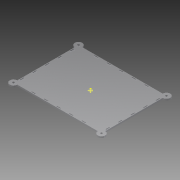
# Autodesk Inventor part: BasePlate2
Saved by Autodesk Inventor 2015 (Build 190159000, 159)
## iProperties
Created: 2014-08-06
Part Number: BasePlate2
Material: Acrylic, Clear
Document SubType Name: Modeling
Designer: Patrick Camilleri
Density: 1.19 g/cm^3
Appearance: Transparent - Clear
Mass: 654.149 g
Surface Area: 1962.87 cm^2
Volume: 549.705 cm^3
Author: Patrick Camilleri
Autodesk Inventor part; units mm, degrees
ref_plane "YZ Plane" through (0, 0, 0) normal (1, 0, 0) x (0, 1, 0)
ref_plane "XZ Plane" through (0, 0, 0) normal (0, 1, 0) x (-1, 0, 0)
ref_plane "XY Plane" through (0, 0, 0) normal (0, 0, 1) x (1, 0, 0)
sketch "Sketch1" plane through (0, 0, 0) normal (0, 0, 1) x (1, 0, 0)
  line L0 (-175, 129.3) -> (175, 129.3)
  line L1 (175, 129.3) -> (175, -129.3)
  line L2 (175, -129.3) -> (-175, -129.3)
  line L3 (-175, -129.3) -> (-175, 129.3)
  line L4 (-175, 129.3) -> (175, -129.3) construction
  line L5 (175, 129.3) -> (-175, -129.3) construction
  circle A0 centre (-175, -129.3) radius 15
  circle A1 centre (-175, 129.3) radius 15
  circle A2 centre (175, 129.3) radius 15
  circle A3 centre (175, -129.3) radius 15
  point P0 (0, 0)
  dimension "d0" = 350
  dimension "d1" = 258.6
  dimension "d2" = 30
  dimension "d3" = 30
  dimension "d4" = 30
  dimension "d5" = 30
  constraints: 12 end point, 4 centre point, 4 coincident, 2 midpoint, 2 parallel, 1 horizontal, 1 perpendicular
  measures "d0" distance of L1.end L2.end
  measures "d1" distance of L0.end L1.end
  measures "d2" diameter of A0
  measures "d3" diameter of A1
  measures "d4" diameter of A2
  measures "d5" diameter of A3
extrude "Extrusion1" add sketch "Sketch1" along normal blind 6
hole "Hole1" at (-175, 129.3, 6) direction (0, 0, -1) diameter 8 end through all
mirror "Mirror1" about plane through (0, 0, 0) normal (1, 0, 0) of "Hole1"
mirror "Mirror2" about plane through (0, 0, 0) normal (0, 1, 0) of "Hole1", "Mirror1"
sketch "Sketch2" plane through (0, 0, 6) normal (0, 0, 1) x (1, 0, 0)
  line L0 (160, 129.3) -> (-160, 129.3) projected
  line L1 (-175, 114.3) -> (-175, -114.3) projected
  line L2 (-160, -129.3) -> (160, -129.3) projected
  line L3 (175, -114.3) -> (175, 114.3) projected
  line L4 (-170.5, 124.8) -> (170.5, 124.8) construction
  line L5 (170.5, 124.8) -> (170.5, -124.8) construction
  line L6 (170.5, -124.8) -> (-170.5, -124.8) construction
  line L7 (-170.5, -124.8) -> (-170.5, 124.8) construction
  line L8 (-170.5, 124.8) -> (170.5, -124.8) construction
  line L9 (170.5, 124.8) -> (-170.5, -124.8) construction
  line L10 (-7.5, 126.3) -> (7.5, 126.3)
  line L11 (7.5, 126.3) -> (7.5, 123.3)
  line L12 (7.5, 123.3) -> (-7.5, 123.3)
  line L13 (-7.5, 123.3) -> (-7.5, 126.3)
  line L14 (-7.5, 126.3) -> (7.5, 123.3) construction
  line L15 (7.5, 126.3) -> (-7.5, 123.3) construction
  line L16 (-57.5, 126.3) -> (-42.5, 126.3)
  line L17 (-42.5, 126.3) -> (-42.5, 123.3)
  line L18 (-42.5, 123.3) -> (-57.5, 123.3)
  line L19 (-57.5, 123.3) -> (-57.5, 126.3)
  line L20 (-107.5, 126.3) -> (-92.5, 126.3)
  line L21 (-92.5, 126.3) -> (-92.5, 123.3)
  line L22 (-92.5, 123.3) -> (-107.5, 123.3)
  line L23 (-107.5, 123.3) -> (-107.5, 126.3)
  line L24 (42.5, 126.3) -> (57.5, 126.3)
  line L25 (57.5, 126.3) -> (57.5, 123.3)
  line L26 (57.5, 123.3) -> (42.5, 123.3)
  line L27 (42.5, 123.3) -> (42.5, 126.3)
  line L28 (92.5, 126.3) -> (107.5, 126.3)
  line L29 (107.5, 126.3) -> (107.5, 123.3)
  line L30 (107.5, 123.3) -> (92.5, 123.3)
  line L31 (92.5, 123.3) -> (92.5, 126.3)
  line L32 (7.5, -126.3) -> (-7.5, -126.3)
  line L33 (-7.5, -126.3) -> (-7.5, -123.3)
  line L34 (-7.5, -123.3) -> (7.5, -123.3)
  line L35 (7.5, -123.3) -> (7.5, -126.3)
  line L36 (7.5, -126.3) -> (-7.5, -123.3) construction
  line L37 (-7.5, -126.3) -> (7.5, -123.3) construction
  line L38 (57.5, -126.3) -> (42.5, -126.3)
  line L39 (42.5, -126.3) -> (42.5, -123.3)
  line L40 (42.5, -123.3) -> (57.5, -123.3)
  line L41 (57.5, -123.3) -> (57.5, -126.3)
  line L42 (107.5, -126.3) -> (92.5, -126.3)
  line L43 (92.5, -126.3) -> (92.5, -123.3)
  line L44 (92.5, -123.3) -> (107.5, -123.3)
  line L45 (107.5, -123.3) -> (107.5, -126.3)
  line L46 (120.5, -124.8) -> (-220.5, -124.8) construction
  line L47 (-42.5, -126.3) -> (-57.5, -126.3)
  line L48 (-57.5, -126.3) -> (-57.5, -123.3)
  line L49 (-57.5, -123.3) -> (-42.5, -123.3)
  line L50 (-42.5, -123.3) -> (-42.5, -126.3)
  line L51 (70.5, -124.8) -> (-270.5, -124.8) construction
  line L52 (-92.5, -126.3) -> (-107.5, -126.3)
  line L53 (-107.5, -126.3) -> (-107.5, -123.3)
  line L54 (-107.5, -123.3) -> (-92.5, -123.3)
  line L55 (-92.5, -123.3) -> (-92.5, -126.3)
  line L56 (-172, 7.5) -> (-169, 7.5)
  line L57 (-169, 7.5) -> (-169, -7.5)
  line L58 (-169, -7.5) -> (-172, -7.5)
  line L59 (-172, -7.5) -> (-172, 7.5)
  line L60 (-172, 7.5) -> (-169, -7.5) construction
  line L61 (-169, 7.5) -> (-172, -7.5) construction
  line L62 (-172, -42.5) -> (-169, -42.5)
  line L63 (-169, -42.5) -> (-169, -57.5)
  line L64 (-169, -57.5) -> (-172, -57.5)
  line L65 (-172, -57.5) -> (-172, -42.5)
  line L66 (-172, -92.5) -> (-169, -92.5)
  line L67 (-169, -92.5) -> (-169, -107.5)
  line L68 (-169, -107.5) -> (-172, -107.5)
  line L69 (-172, -107.5) -> (-172, -92.5)
  line L70 (-172, 57.5) -> (-169, 57.5)
  line L71 (-169, 57.5) -> (-169, 42.5)
  line L72 (-169, 42.5) -> (-172, 42.5)
  line L73 (-172, 42.5) -> (-172, 57.5)
  line L74 (-172, 107.5) -> (-169, 107.5)
  line L75 (-169, 107.5) -> (-169, 92.5)
  line L76 (-169, 92.5) -> (-172, 92.5)
  line L77 (-172, 92.5) -> (-172, 107.5)
  line L78 (169, 7.5) -> (172, 7.5)
  line L79 (172, 7.5) -> (172, -7.5)
  line L80 (172, -7.5) -> (169, -7.5)
  line L81 (169, -7.5) -> (169, 7.5)
  line L82 (169, 7.5) -> (172, -7.5) construction
  line L83 (172, 7.5) -> (169, -7.5) construction
  line L84 (169, 57.5) -> (172, 57.5)
  line L85 (172, 57.5) -> (172, 42.5)
  line L86 (172, 42.5) -> (169, 42.5)
  line L87 (169, 42.5) -> (169, 57.5)
  line L88 (169, 107.5) -> (172, 107.5)
  line L89 (172, 107.5) -> (172, 92.5)
  line L90 (172, 92.5) -> (169, 92.5)
  line L91 (169, 92.5) -> (169, 107.5)
  line L92 (169, -42.5) -> (172, -42.5)
  line L93 (172, -42.5) -> (172, -57.5)
  line L94 (172, -57.5) -> (169, -57.5)
  line L95 (169, -57.5) -> (169, -42.5)
  line L96 (169, -92.5) -> (172, -92.5)
  line L97 (172, -92.5) -> (172, -107.5)
  line L98 (172, -107.5) -> (169, -107.5)
  line L99 (169, -107.5) -> (169, -92.5)
  point P0 (0, 0)
  point P1 (0, 124.8)
  point P2 (0, -124.8)
  point P3 (-50, -124.8)
  point P4 (-100, -124.8)
  point P5 (-170.5, 0)
  point P6 (170.5, 0)
  dimension "d44" = 4.5
  dimension "d45" = 4.5
  dimension "d46" = 15
  dimension "d47" = 3
  dimension "d50" = 50
  dimension "d57" = 50
  dimension "d62" = 3
  dimension "d65" = 50
  dimension "d72" = 50
  dimension "d77" = 3
  dimension "d78" = 15
  dimension "d81" = 50
  dimension "d88" = 50
  dimension "d95" = 50
  dimension "d102" = 50
  dimension "d109" = 15
  dimension "d110" = 15
  constraints: 192 end point, 14 midpoint, 10 parallel, 9 horizontal, 5 perpendicular, 4 vertical, 136 other
  measures "d44" distance between parallel lines of L3 L5
  measures "d45" distance between parallel lines of L0 L4
  measures "d46" distance of L11.end L12.end
  measures "d47" distance of L10.end L11.end
  measures "d50" distance of L10.start L16.start
  measures "d57" distance of L11.end L26.start
  measures "d62" distance of L33.end L32.end
  measures "d65" distance of L32.start L38.start
  measures "d72" distance of L34.end L50.start
  measures "d77" distance of L57.end L58.end
  measures "d78" distance of L56.end L57.end
  measures "d81" distance of L57.end L64.start
  measures "d88" distance of L56.end L71.start
  measures "d95" distance of L79.end L86.start
  measures "d102" distance of L78.start L92.start
  measures "d109" distance of L80.end L78.start
  measures "d110" distance of L32.start L32.end
extrude "Extrusion2" cut sketch "Sketch2" against normal blind 6
equation "\"d3\" = d2"
equation "\"d4\" = d2"
equation "\"d5\" = d2"
body "Solid1"
